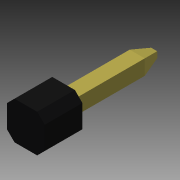
# Autodesk Inventor part: nanopc_t4_pin
Saved by Autodesk Inventor 2013 SP2 (Build 170200200, 200)
## iProperties
Created: 2018-09-03
Part Number: nanopc_t4_pin
Material: Generic
Document SubType Name: Modeling
Designer: alex
Density: 1 g/cm^3
Author: alex
Autodesk Inventor part; units mm, degrees
ref_plane "YZ Plane" through (0, 0, 0) normal (1, 0, 0) x (0, 1, 0)
ref_plane "XZ Plane" through (0, 0, 0) normal (0, 1, 0) x (-1, 0, 0)
ref_plane "XY Plane" through (0, 0, 0) normal (0, 0, 1) x (1, 0, 0)
sketch "Sketch1" plane through (0, 0, 0) normal (0, 1, 0) x (-1, 0, 0)
  line L0 (-1.25, -1.25) -> (1.25, -1.25)
  line L1 (1.25, -1.25) -> (1.25, 1.25)
  line L2 (1.25, 1.25) -> (-1.25, 1.25)
  line L3 (-1.25, 1.25) -> (-1.25, -1.25)
  line L4 (-1.25, -1.25) -> (1.25, 1.25) construction
  line L5 (1.25, -1.25) -> (-1.25, 1.25) construction
  point P0 (0, 0)
  dimension "d0" = 2.5
  dimension "d1" = 2.5
  constraints: 12 end point, 2 midpoint, 2 parallel, 1 horizontal, 1 perpendicular
  measures "d0" distance of L2.end L1.end
  measures "d1" distance of L1.end L0.end
extrude "Extrusion1" add sketch "Sketch1" along normal blind 2.5
chamfer "Chamfer1" distance 0.5 angle 45 4 edges at (1.25, 1.25, 1.25) (-1.25, 1.25, 1.25) (1.25, 1.25, -1.25) (-1.25, 1.25, -1.25)
sketch "Sketch2" plane through (0, 2.5, 0) normal (0, 1, 0) x (1, 0, 0)
  line L0 (-0.5, 0.5) -> (0.5, 0.5)
  line L1 (0.5, 0.5) -> (0.5, -0.5)
  line L2 (0.5, -0.5) -> (-0.5, -0.5)
  line L3 (-0.5, -0.5) -> (-0.5, 0.5)
  point P0 (0, 0)
  dimension "d7" = 1
  dimension "d9" = 1
  dimension "d10" = 0.5
  dimension "d11" = 0.5
  constraints: 8 end point, 2 parallel, 1 horizontal, 1 perpendicular
  measures "d7" distance of L1.end L2.end
  measures "d9" distance of L0.end L1.end
  measures "d10" distance from line of L0 point (0, 0)
  measures "d11" distance from line of L3 point (0, 0)
extrude "Extrusion2" add sketch "Sketch2" along normal blind 6
chamfer "Chamfer2" distance 0.3 angle 75 4 edges at (0, 8.5, 0.5) (-0.5, 8.5, 0) (0, 8.5, -0.5) (0.5, 8.5, 0) measured on face at (-0.1667, 8.5, -0.1667)
body "Solid1"
